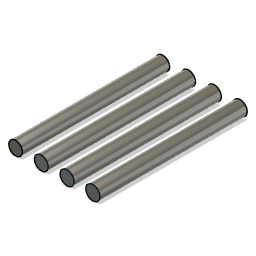
Hinge+Rods (Autodesk Fusion 360 design; units mm, degrees)
Autodesk Fusion 360 part; units mm, degrees
sketch "Sketch1" plane through (0, 0, 0) normal (0, 0, 1) x (1, 0, 0)
  circle A0 centre (0, 0) radius 3.175
  dimension "d1" = 6.35
  constraint coincident A0.centre origin
  measures "d1" diameter of A0
extrude "Extrude1" add sketch "Sketch1" along normal blind 101.6 makes body 1
copy_body "CopyPasteBodies1" bodies 1 makes body 2
move_body "Move1" bodies 2 to x (1, 0, 0) y (0, 1, 0) z (0, 0, 1) at (17.78, 0, 0)
copy_body "CopyPasteBodies2" bodies 2 1 makes body 3 makes body 4
move_body "Move2" bodies 3 4 to x (1, 0, 0) y (0, 1, 0) z (0, 0, 1) at (35.56, 0, 0)
move_face "OffsetFaces1" offset 1.524 1 faces at (3.1592, -0.3161, 67.7333) on bodies 1
move_face "OffsetFaces2" offset 1.5875 1 faces at (20.9392, -0.3161, 67.7333) on bodies 2
move_face "OffsetFaces3" offset 1.651 1 faces at (38.7192, -0.3161, 67.7333) on bodies 4
move_face "OffsetFaces4" offset 1.7145 1 faces at (56.4992, -0.3161, 67.7333) on bodies 3
sketch "Sketch2" plane through (0, 0, 101.6) normal (0, 0, 1) x (1, 0, 0)
  circle A0 centre (53.34, 0) radius 4.8895
sketch "Sketch3" plane through (0, 0, 101.6) normal (0, 0, 1) x (1, 0, 0)
  circle A0 centre (35.56, 0) radius 4.826
sketch "Sketch4" plane through (0, 0, 101.6) normal (0, 0, 1) x (1, 0, 0)
  circle A0 centre (17.78, 0) radius 4.7625
